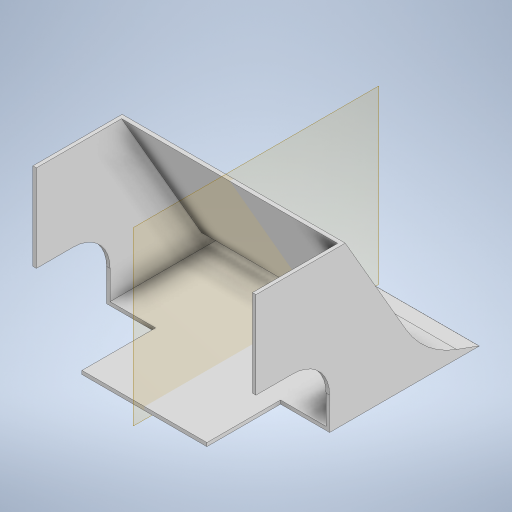
# Autodesk Inventor part: Body
Saved by Autodesk Inventor 2024 (Build 280153000, 153)
## iProperties
Created: 2023-10-20
Part Number: Body
Material: Generic
Document SubType Name: Modeling
Designer: kdcao
Density: 1 g/cm^3
Appearance: Default
Author: kdcao
Autodesk Inventor part; units mm, degrees
ref_plane "YZ Plane" through (0, 0, 0) normal (1, 0, 0) x (0, 1, 0)
ref_plane "XZ Plane" through (0, 0, 0) normal (0, 1, 0) x (-1, 0, 0)
ref_plane "XY Plane" through (0, 0, 0) normal (0, 0, 1) x (1, 0, 0)
sketch "Sketch1" plane through (0, 0, 0) normal (0, 1, 0) x (-1, 0, 0)
  line L0 (-50, 50) -> (50, 50)
  line L1 (50, 50) -> (50, -50)
  line L2 (50, -50) -> (-50, -50)
  line L3 (-50, -50) -> (-50, 50)
  line L4 (-50, 50) -> (50, -50) construction
  line L5 (50, 50) -> (-50, -50) construction
  point P0 (0, 0)
  dimension "d0" = 100
  dimension "d1" = 100
  constraints: 12 end point, 2 midpoint, 2 parallel, 1 horizontal, 1 perpendicular
  measures "d0" distance of L0.end L1.end
  measures "d1" distance of L1.end L2.end
extrude "Extrusion1" add sketch "Sketch1" along normal blind 70
sketch "Sketch2" plane through (50, 0, 50) normal (1, 0, 0) x (0, 0, -1)
  line L0 (100, 0) -> (100, 70) projected
  line L1 (100, 0.1) -> (75.1308, 9.1516)
  line L2 (75.1308, 9.1516) -> (40, 70)
  line L3 (100, 70) -> (0, 70) projected
  line L4 (100, 70) -> (100, 0.1)
  line L5 (0, 0) -> (100, 0) projected
  point P0 (50, 0)
  dimension "d4" = 20
  dimension "d5" = 60
  dimension "d6" = 0.1
  dimension "d9" = 40
  constraints: 6 end point, 2 point on line, 1 vertical
  measures "d4" angle of L5 L1
  measures "d5" angle of L3 L2
  measures "d6" distance of L0.start L1.start
  measures "d9" distance of L3.end L2.end
extrude "Extrusion2" cut sketch "Sketch2" against normal through all
shell "Shell1" thickness 1.5875 removed faces 1 at (16.6667, 70, 36.6667)
shell "Shell2" thickness 1.5875 removed faces 3 at (-16.1375, 47.1958, 48.4125) at (-16.6667, 23.3333, 50) at (16.1375, 70, 10.611)
sketch "Sketch3" plane through (50, 0, 50) normal (1, 0, 0) x (0, 0, -1)
  circle A0 centre (16.5, 14.5) radius 16.5
  line L0 (0, 0) -> (0, 70) projected
  line L1 (0, 0) -> (100, 0) projected
  line L2 (0, 14.5) -> (0, 0)
  line L3 (0, 0) -> (33, 0)
  line L4 (33, 14.5) -> (33, 0)
  line L5 (91.2716, 1.5875) -> (0, 1.5875) projected
  line L6 (16.5, 31) -> (0, 31)
  point P0 (50, 0)
  point P1 (98.4125, 1.5875)
  dimension "d12" = 33
  dimension "d13" = 16.5
  dimension "d14" = 14.5
  constraints: 8 end point, 3 point on circle, 3 point on line, 2 perpendicular, 1 centre point, 1 collinear, 1 tangent
  measures "d12" diameter of A0
  measures "d13" distance from line of L0 A0.centre
  measures "d14" distance from line of L1 A0.centre
extrude "Extrusion3" cut sketch "Sketch3" against normal blind 22 contours A0 L5 | L4 L5 A0 | A0 L0 L6 | L5 L4 L1 A0 | A0 L1 L5 | A0 L5 L0 | A0 L1 L0 L5
ref_plane "Work Plane1" through (0, 0, -50) normal (1, 0, 0) x (0, 0, -1)
mirror "Mirror1" about plane through (0, 0, -50) normal (1, 0, 0) of "Extrusion3"
fillet "Fillet1" radius 43.275 1 edges at (0, 9.1516, -25.1308)
body "Solid1"
